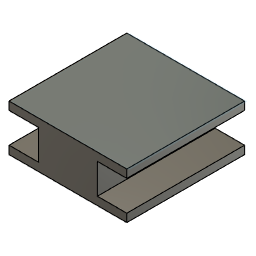
half_inch_armor_spacers (Autodesk Fusion 360 design; units mm, degrees)
Autodesk Fusion 360 part; units mm, degrees
sketch "Sketch1" plane through (0, 0, 0) normal (0, 1, 0) x (1, 0, 0)
  line L0 (0, 0) -> (25.4, 0)
  line L1 (25.4, 0) -> (25.4, -25.4)
  line L2 (25.4, -25.4) -> (0, -25.4)
  line L3 (0, -25.4) -> (0, 0)
  dimension "d1" = 25.4
  dimension "d2" = 25.4
  constraint horizontal L0
  constraint vertical L1
  constraint horizontal L2
  constraint vertical L3
  constraint coincident L0.start L3.end
  measures "d1" distance of L0.start L0.end
  measures "d2" distance of L0.start L2.end
extrude "Extrude1" add sketch "Sketch1" along normal blind 10 makes body 1
sketch "Sketch2" plane through (0, 10, 0) normal (0, 1, 0) x (-1, 0, 0)
  line L0 (0, 25.4) -> (-25.4, 25.4)
  line L1 (-25.4, 25.4) -> (-25.4, 0)
  line L2 (-25.4, 0) -> (0, 0)
  line L3 (0, 0) -> (0, 25.4)
sketch "Sketch3" plane through (0, 0, 0) normal (-1, 0, 0) x (0, 0, 1)
  line L0 (0, 0) -> (25.4, 0)
  line L1 (25.4, 0) -> (25.4, 10)
  line L2 (25.4, 10) -> (0, 10)
  line L3 (0, 10) -> (0, 0)
  line L4 (0, 10) -> (25.4, 10)
  line L5 (25.4, 10) -> (25.4, 8.25)
  line L6 (25.4, 8.25) -> (0, 8.25)
  line L7 (0, 8.25) -> (0, 10)
  line L8 (0, 0) -> (25.4, 0)
  line L9 (25.4, 0) -> (25.4, 1.75)
  line L10 (25.4, 1.75) -> (0, 1.75)
  line L11 (0, 1.75) -> (0, 0)
  dimension "d5" = 1.75
  dimension "d6" = 1.75
  constraint horizontal L4
  constraint vertical L5
  constraint horizontal L6
  constraint vertical L7
  constraint coincident L2.end L3.start
  constraint horizontal L8
  constraint vertical L9
  constraint horizontal L10
  constraint vertical L11
  constraint coincident L1 L9.end
  constraint coincident L0.start L3.end
  measures "d5" distance of L2.end L6.end
  measures "d6" distance of L0.start L10.end
extrude "Extrude2" cut sketch "Sketch3" against normal blind 6.35 contours L1 L3 L6 L10 bodies 1
sketch "Sketch4" plane through (25.4, 0, 0) normal (1, 0, 0) x (0, 0, -1)
  line L0 (-25.4, 0) -> (0, 0)
  line L1 (0, 0) -> (0, 10)
  line L2 (0, 10) -> (-25.4, 10)
  line L3 (-25.4, 10) -> (-25.4, 0)
  line L4 (-25.4, 10) -> (0, 10)
  line L5 (0, 10) -> (0, 8.25)
  line L6 (0, 8.25) -> (-25.4, 8.25)
  line L7 (-25.4, 8.25) -> (-25.4, 10)
  line L8 (-25.4, 0) -> (0, 0)
  line L9 (0, 0) -> (0, 1.75)
  line L10 (0, 1.75) -> (-25.4, 1.75)
  line L11 (-25.4, 1.75) -> (-25.4, 0)
  dimension "d9" = 1.75
  dimension "d10" = 25.4
  dimension "d11" = 1.75
  constraint horizontal L4
  constraint vertical L5
  constraint horizontal L6
  constraint vertical L7
  constraint coincident L2.end L3.start
  constraint horizontal L8
  constraint vertical L9
  constraint horizontal L10
  constraint vertical L11
  constraint coincident L0.start L3.end
  measures "d9" distance of L2.end L6.end
  measures "d10" distance of L0.start L0.end
  measures "d11" distance of L0.start L10.end
extrude "Extrude3" cut sketch "Sketch4" against normal blind 6.35 contours L1 L3 L6 L10 bodies 1
copy_body "Body->Comp1" bodies 1 removing the originals makes body 2 in component "Half inch spacer"
component "Half inch spacer" placed x (1, 0, 0) y (0, 1, 0) z (0, 0, 1) at (0, 0, 0)
